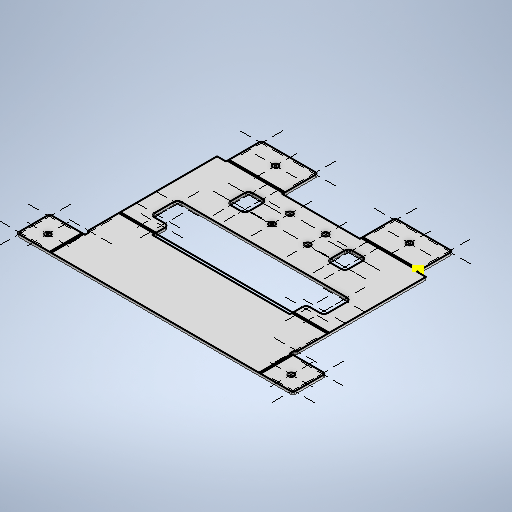
# Autodesk Inventor part: body_top_frame
Saved by Autodesk Inventor 2026.1 (Build 301233000, 233)
## iProperties
Created: 2025-08-22
Part Number: body_top_frame
Material: Generic
Document SubType Name: Modeling
Designer: chris
Density: 1 g/cm^3
Appearance: Default
Author: chris
Autodesk Inventor part; units mm, degrees
ref_plane "YZ Plane" through (0, 0, 0) normal (1, 0, 0) x (0, 1, 0)
ref_plane "XZ Plane" through (0, 0, 0) normal (0, 1, 0) x (-1, 0, 0)
ref_plane "XY Plane" through (0, 0, 0) normal (0, 0, 1) x (1, 0, 0)
sketch "Sketch1" plane through (0, 0, 0) normal (0, 1, 0) x (-1, 0, 0)
  line L0 (-5, 55.3296) -> (112, 55.3296)
  line L1 (75.5, -0.4496) -> (107, -0.4496)
  line L2 (-5.1396, 93.9693) -> (-5.1396, 75.7793)
  line L3 (112.1396, 75.7793) -> (112.1396, 93.9693)
  line L4 (0, -0.4496) -> (32, -0.4496)
  arc A0 (30.54, 18.62) -> (28.54, 20.62) centre (28.54, 18.62) ccw
  line L5 (22.54, 20.62) -> (28.54, 20.62)
  arc A1 (28.54, 8.62) -> (30.54, 10.62) centre (28.54, 10.62) ccw
  line L6 (30.54, 18.62) -> (30.54, 10.62)
  arc A2 (22.54, 20.62) -> (20.54, 18.62) centre (22.54, 18.62) ccw
  line L7 (20.54, 10.62) -> (20.54, 18.62)
  arc A3 (20.54, 10.62) -> (22.54, 8.62) centre (22.54, 10.62) ccw
  line L8 (28.54, 8.62) -> (22.54, 8.62)
  arc A4 (78.46, 20.62) -> (76.46, 18.62) centre (78.46, 18.62) ccw
  line L9 (76.46, 10.62) -> (76.46, 18.62)
  arc A5 (86.46, 18.62) -> (84.46, 20.62) centre (84.46, 18.62) ccw
  line L10 (78.46, 20.62) -> (84.46, 20.62)
  arc A6 (76.46, 10.62) -> (78.46, 8.62) centre (78.46, 10.62) ccw
  line L11 (84.46, 8.62) -> (78.46, 8.62)
  arc A7 (84.46, 8.62) -> (86.46, 10.62) centre (84.46, 10.62) ccw
  line L12 (86.46, 18.62) -> (86.46, 10.62)
  arc A8 (7, 47.88) -> (5, 45.88) centre (7, 45.88) ccw
  line L13 (5, 34.88) -> (5, 45.88)
  arc A9 (13, 47.88) -> (15, 49.88) centre (13, 49.88) ccw
  line L14 (15, 49.88) -> (15, 56.9693)
  arc A10 (5, 34.88) -> (7, 32.88) centre (7, 34.88) ccw
  line L15 (100, 32.88) -> (7, 32.88)
  arc A11 (92, 49.88) -> (94, 47.88) centre (94, 49.88) ccw
  line L16 (92, 56.9693) -> (92, 49.88)
  arc A12 (102, 45.88) -> (100, 47.88) centre (100, 45.88) ccw
  line L17 (94, 47.88) -> (100, 47.88)
  arc A13 (100, 32.88) -> (102, 34.88) centre (100, 34.88) ccw
  line L18 (102, 45.88) -> (102, 34.88)
  line L19 (15, 56.9693) -> (92, 56.9693)
  line L20 (7, 47.88) -> (13, 47.88)
  circle A14 centre (91, -10.9943) radius 1.55
  circle A15 centre (16, -10.9943) radius 1.55
  circle A16 centre (121.6843, 85.8743) radius 1.55
  circle A17 centre (-14.6843, 85.8743) radius 1.55
  circle A18 centre (63.75, 8.19) radius 1.55
  circle A19 centre (63.75, 18.19) radius 1.55
  circle A20 centre (43.75, 8.19) radius 1.55
  circle A21 centre (43.75, 18.19) radius 1.55
  arc A22 (112, 72.7793) -> (111, 73.7793) centre (111, 72.7793) ccw
  arc A23 (-4, 73.7793) -> (-5, 72.7793) centre (-4, 72.7793) ccw
  line L21 (-3.94, 73.7793) -> (-4, 73.7793)
  arc A24 (-23.7793, 76.7793) -> (-22.7793, 75.7793) centre (-22.7793, 76.7793) ccw
  arc A25 (-22.7793, 93.9693) -> (-23.7793, 92.9693) centre (-22.7793, 92.9693) ccw
  line L22 (-22.7793, 93.9693) -> (129.7793, 93.9693)
  arc A26 (130.7793, 92.9693) -> (129.7793, 93.9693) centre (129.7793, 92.9693) ccw
  arc A27 (129.7793, 75.7793) -> (130.7793, 76.7793) centre (129.7793, 76.7793) ccw
  line L23 (129.7793, 75.7793) -> (110.94, 75.7793)
  arc A28 (31, -19.0893) -> (32, -18.0893) centre (31, -18.0893) ccw
  arc A29 (0, -18.0893) -> (1, -19.0893) centre (1, -18.0893) ccw
  arc A30 (106, -19.0893) -> (107, -18.0893) centre (106, -18.0893) ccw
  arc A31 (75.5, -18.0893) -> (76.5, -19.0893) centre (76.5, -18.0893) ccw
  line L24 (75.5, -18.0893) -> (75.5, 0.75)
  line L25 (106, -19.0893) -> (76.5, -19.0893)
  line L26 (107, 0.75) -> (107, -18.0893)
  line L27 (107, 0.75) -> (112, 0.75)
  line L28 (112, 72.7793) -> (112, 0.75)
  line L29 (31, -19.0893) -> (1, -19.0893)
  line L30 (0, -18.0893) -> (0, 0.75)
  line L31 (-5, 0.75) -> (0, 0.75)
  line L32 (32, 0.75) -> (32, -18.0893)
  line L33 (32, 0.75) -> (75.5, 0.75)
  line L34 (-5, 0.75) -> (-5, 72.7793)
  line L35 (130.7793, 92.9693) -> (130.7793, 76.7793)
  line L36 (-23.7793, 76.7793) -> (-23.7793, 92.9693)
  line L37 (-3.94, 75.7793) -> (-22.7793, 75.7793)
  line L38 (-3.94, 75.7793) -> (-3.94, 73.7793)
  line L39 (111, 73.7793) -> (110.94, 73.7793)
  line L40 (110.94, 73.7793) -> (110.94, 75.7793)
  line L41 (112.5893, 93.9693) -> (112.5893, 75.7793)
  line L42 (-5.5893, 75.7793) -> (-5.5893, 93.9693)
  line L43 (111.69, 75.7793) -> (111.69, 93.9693)
  line L44 (-4.69, 93.9693) -> (-4.69, 75.7793)
  line L45 (32, -0.8993) -> (0, -0.8993)
  line L46 (107, -0.8993) -> (75.5, -0.8993)
  line L47 (-5, 55.7793) -> (15, 55.7793)
  line L48 (92, 55.7793) -> (112, 55.7793)
  line L49 (0, 0) -> (32, 0)
  line L50 (75.5, 0) -> (107, 0)
  line L51 (15, 54.88) -> (-5, 54.88)
  line L52 (112, 54.88) -> (92, 54.88)
  constraints: 106 end point, 57 tangent, 48 point on circle, 34 point on line, 32 centre point, 29 equal radius, 29 horizontal, 24 perpendicular, 24 vertical, 23 parallel, 159 other
extrude "Extrusion1" add sketch "Sketch1" against normal blind 1.5 contours L34 L47 L14 L0 | L0 L14 L51 L34 | L51 L14 A9 L20 A8 L13 A10 L15 A13 L18 A12 L17 A11 L16 L52 L28 L27 L26 L50 L24 L33 L32 L49 L30 L31 L34 | L34 A23 L21 L38 L37 L44 L22 L43 L23 L40 L39 A22 L28 L48 L16 L19 L14 L47 | L16 L48 L28 L0 | L0 L28 L52 L16 | L49 L32 L4 L30 | L4 L32 L45 L30 | L45 L32 A28 L29 A29 L30 | L37 L2 L22 L44 | L26 L1 L24 L50 | L37 L42 L22 L2 | L26 L46 L24 L1 | L37 A24 L36 A25 L22 L42 | L22 L3 L23 L43 | L26 A30 L25 A31 L24 L46 | L22 L41 L23 L3 | L22 A26 L35 A27 L23 L41
body "Solid1"
